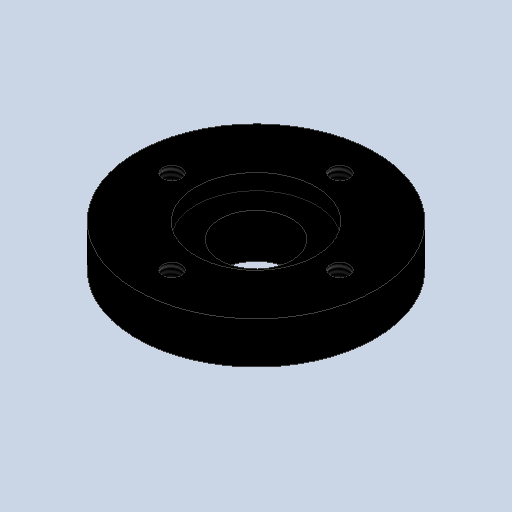
# Autodesk Inventor part: Bottom Horn
Saved by Autodesk Inventor 2026.1 (Build 301233000, 233)
## iProperties
Created: 2022-09-18
Part Number: Bottom Horn
Material: Aluminum 6061-AHC
Document SubType Name: Modeling
Designer: 박동준
Density: 3.171 g/cm^3
Appearance: Aluminum - Dark
Mass: 2.99919 g
Surface Area: 9.91253 cm^2
Volume: 0.945819 cm^3
품번: 7
Author: 박동준
Autodesk Inventor part; units mm, degrees
ref_plane "YZ Plane" through (0, 0, 0) normal (1, 0, 0) x (0, 1, 0)
ref_plane "XZ Plane" through (0, 0, 0) normal (0, 1, 0) x (-1, 0, 0)
ref_plane "XY Plane" through (0, 0, 0) normal (0, 0, 1) x (1, 0, 0)
sketch "스케치1" plane through (0, 0, 0) normal (0, 0, 1) x (1, 0, 0)
  line L0 (0, 6.4532) -> (0, -6.4532)
  line L1 (3, -3.68) -> (3, 0)
  line L2 (3, 0) -> (5, 0)
  line L3 (5, 0) -> (5, 1.32)
  line L4 (5, 1.32) -> (9.96, 1.32)
  line L5 (9.96, 1.32) -> (9.96, -2.16)
  line L6 (9.96, -2.16) -> (4.48, -2.16)
  line L7 (4.48, -2.16) -> (4.48, -3.68)
  line L8 (4.48, -3.68) -> (3, -3.68)
  point P0 (0, 0)
  point P1 (0, 0)
  dimension "d22" = 6
  dimension "d23" = 8.96
  dimension "d24" = 10
  dimension "d25" = 19.92
  dimension "d26" = 1.32
  dimension "d27" = 5
  dimension "d28" = 3.48
  constraints: 18 end point, 7 perpendicular, 2 vertical, 1 coincident, 1 horizontal alignment, 1 midpoint
  measures "d22" diameter of L1 L0
  measures "d23" diameter of L7 L0
  measures "d24" diameter of L3 L0
  measures "d25" diameter of L5 L0
  measures "d26" distance between parallel lines of L2 L4
  measures "d27" distance between parallel lines of L4 L8
  measures "d28" distance between parallel lines of L4 L6
revolve "회전1" add sketch "스케치1" angle 360 about axis through (0, 6.4532, 0) along (0, -1, 0)
sketch "Sketch3" plane through (0, 1.32, 0) normal (0, 1, 0) x (1, 0, 0)
  point P0 (0, 0)
  point P1 (7, 0)
  point P2 (0, 7)
  point P3 (-7, 0)
  point P4 (0, -7)
  dimension "d29" = 7
  dimension "d32" = 360
  constraints: 1 horizontal alignment, 5 other
  measures "d29" distance of point (7, 0) point (0, 0)
hole "Hole2" at (7, 1.32, 0) at (0, 1.32, -7) at (-7, 1.32, 0) at (0, 1.32, 7) direction (0, -1, 0) diameter 1.567 end through all thread size "M2x0.4" class "6H" standard "ISO Metric profile"
